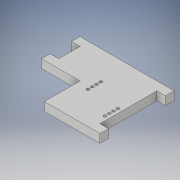
# Autodesk Inventor part: thumper-bumper-sidewall3-v2
Saved by Autodesk Inventor 2017 (Build 210142000, 142)
## iProperties
Created: 2017-02-22
Part Number: thumper-bumper-sidewall3-v2
Material: Generic
Document SubType Name: Modeling
Designer: John
Density: 1 g/cm^3
Appearance: Default
Author: John
Autodesk Inventor part; units mm, degrees
ref_plane "YZ Plane" through (0, 0, 0) normal (1, 0, 0) x (0, 1, 0)
ref_plane "XZ Plane" through (0, 0, 0) normal (0, 1, 0) x (-1, 0, 0)
ref_plane "XY Plane" through (0, 0, 0) normal (0, 0, 1) x (1, 0, 0)
sketch "Sketch1" plane through (0, 0, 0) normal (0, 1, 0) x (-1, 0, 0)
  line L0 (0, 0) -> (60, 0)
  line L1 (66, 0) -> (66, 6)
  line L2 (66, 27) -> (60, 27)
  line L3 (0, 27) -> (0, 6) construction
  line L4 (66, 27) -> (60, 27)
  line L5 (60, 27) -> (60, 21) construction
  line L6 (60, 21) -> (66, 21)
  line L7 (66, 21) -> (66, 27)
  line L8 (66, 0) -> (60, 0)
  line L9 (60, 0) -> (60, 6) construction
  line L10 (60, 6) -> (66, 6)
  line L11 (66, 6) -> (66, 0)
  line L12 (66, 21) -> (66, 27)
  line L13 (60, 27) -> (6, 27)
  line L14 (60, 0) -> (66, 0)
  line L15 (66, 6) -> (66, 21) construction
  line L16 (60, 6) -> (60, 21)
  line L17 (0, 0) -> (6, 0)
  line L18 (6, 0) -> (6, 6) construction
  line L19 (6, 6) -> (0, 6)
  line L20 (0, 6) -> (0, 0)
  line L21 (6, 6) -> (6, 27)
  line L22 (6, 27) -> (0, 27) construction
  line L23 (0, 6) -> (0, 0)
  line L24 (6, 27) -> (39, 27)
  line L25 (39, 27) -> (39, 52)
  line L26 (39, 52) -> (6, 52)
  line L27 (6, 52) -> (0, 52)
  line L28 (0, 52) -> (0, 46)
  line L29 (0, 46) -> (6, 46)
  line L30 (6, 46) -> (6, 52) construction
  line L31 (6, 46) -> (6, 27)
  dimension "d0" = 66
  dimension "d1" = 27
  dimension "d2" = 6
  dimension "d3" = 6
  dimension "d4" = 6
  dimension "d5" = 6
  dimension "d6" = 6
  dimension "d7" = 6
  dimension "d10" = 33
  dimension "d11" = 25
  dimension "d12" = 6
  dimension "d13" = 6
  constraints: 64 end point, 22 parallel, 13 perpendicular, 7 horizontal
  measures "d0" distance of L3.start L2.start
  measures "d1" distance of L2.start L1.start
  measures "d2" distance of L6.end L5.end
  measures "d3" distance of L5.end L2.end
  measures "d4" distance of L9.end L1.end
  measures "d5" distance of L0.end L9.end
  measures "d6" distance of L3.end L18.end
  measures "d7" distance of L18.end L17.end
  measures "d10" distance of L26.end L25.end
  measures "d11" distance of L25.end L24.end
  measures "d12" distance of L29.end L28.end
  measures "d13" distance of L28.end L27.end
extrude "Extrusion1" add sketch "Sketch1" along normal blind 6
sketch "Sketch2" plane through (0, 6, 0) normal (0, 1, 0) x (1, 0, 0)
  circle A0 centre (-8.9, -39.536) radius 1
  line L0 (0, -46) -> (-6, -46) projected
  line L1 (-6, -46) -> (-6, -6) projected
  circle A1 centre (-31.1, -29.236) radius 1
  circle A2 centre (-8.9, -36.536) radius 1
  circle A3 centre (-8.9, -33.536) radius 1
  circle A4 centre (-8.9, -30.536) radius 1
  circle A5 centre (-31.1, -26.236) radius 1
  circle A6 centre (-31.1, -23.236) radius 1
  circle A7 centre (-31.1, -20.236) radius 1
  point P0 (0, 0)
  dimension "d14" = 2
  dimension "d15" = 6.464
  dimension "d16" = 2.9
  dimension "d19" = 2
  dimension "d20" = 22.2
  dimension "d21" = 10.3
  dimension "d22" = 2
  dimension "d23" = 3
  dimension "d24" = 2
  dimension "d25" = 3
  dimension "d26" = 2
  dimension "d27" = 3
  dimension "d28" = 2
  dimension "d29" = 2
  dimension "d30" = 3
  dimension "d31" = 2
  dimension "d32" = 3
  dimension "d33" = 3
  constraints: 8 centre point
  measures "d14" diameter of A0
  measures "d15" distance from line of L0 A0.centre
  measures "d16" distance from line of L1 A0.centre
  measures "d19" diameter of A1
  measures "d20" horizontal distance of A1.centre A0.centre
  measures "d21" vertical distance of A1.centre A0.centre
  measures "d22" diameter of A2
  measures "d23" distance of A0.centre A2.centre
  measures "d24" diameter of A3
  measures "d25" distance of A3.centre A2.centre
  measures "d26" diameter of A4
  measures "d27" distance of A4.centre A3.centre
  measures "d28" diameter of A5
  measures "d29" diameter of A6
  measures "d30" distance of A6.centre A5.centre
  measures "d31" diameter of A7
  measures "d32" distance of A7.centre A6.centre
  measures "d33" distance of A5.centre A1.centre
extrude "Extrusion2" cut sketch "Sketch2" against normal through all
body "Solid1"
